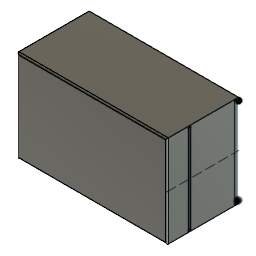
Control board - base v4 (Autodesk Fusion 360 design; units mm, degrees)
Autodesk Fusion 360 part; units mm, degrees
sketch "Esquisse1" plane through (0, 0, 0) normal (0, 1, 0) x (1, 0, 0)
  line L0 (-41.4317, -0.2961) -> (62.5683, -0.2961)
  line L1 (62.5683, -0.2961) -> (62.5683, -64.2961)
  line L2 (62.5683, -64.2961) -> (-41.4317, -64.2961)
  line L3 (-41.4317, -64.2961) -> (-41.4317, -0.2961)
  dimension "d1" = 104
  dimension "d2" = 64
  constraint horizontal L0
  constraint vertical L1
  constraint horizontal L2
  constraint vertical L3
  measures "d1" distance of L1 L3
  measures "d2" distance of L0 L2
extrude "Extrusion1" add sketch "Esquisse1" along normal blind 50
shell "Coque1" thickness 2 removed faces 1 at (-6.765, 50, 21.6294)
sketch "Sketch4" plane through (62.5683, 0, 0) normal (1, 0, 0) x (0, 1, 0)
  line L0 (0, 64.2961) -> (0, 0.2961)
  line L1 (0, 0.2961) -> (50, 0.2961)
  line L2 (50, 0.2961) -> (50, 64.2961)
  line L3 (50, 64.2961) -> (0, 64.2961)
  line L4 (0, 32.2961) -> (50, 32.2961) construction
  line L5 (15, 63.3961) -> (16.4, 63.3961)
  line L6 (16.4, 63.3961) -> (16.4, 1.1961)
  line L7 (16.4, 1.1961) -> (15, 1.1961)
  line L8 (15, 1.1961) -> (15, 63.3961)
  line L9 (48.8, 1.1961) -> (47.4, 1.1961)
  line L10 (47.4, 1.1961) -> (47.4, 63.3961)
  line L11 (47.4, 63.3961) -> (48.8, 63.3961)
  line L12 (48.8, 63.3961) -> (48.8, 1.1961)
  line L13 (48.8, 62.2961) -> (50, 62.2961)
  line L14 (48.8, 2.2961) -> (50, 2.2961)
  dimension "d19" = 1.4
  dimension "d20" = 1.4
  dimension "d55" = 31
  dimension "d66" = 0.9
  dimension "d67" = 2
  dimension "d79" = 15
  constraint midpoint L0 L4.start
  constraint midpoint L2 L4.end
  constraint horizontal L5
  constraint vertical L6
  constraint horizontal L7
  constraint vertical L8
  constraint symmetric L4 L5 L7
  constraint horizontal L9
  constraint vertical L10
  constraint horizontal L11
  constraint vertical L12
  constraint symmetric L4 L9 L11
  constraint collinear L5 L11
  constraint coincident L12 L13.start
  constraint coincident L2 L13.end
  constraint perpendicular L2 L13
  constraint symmetric L4 L13.start L14.start
  constraint symmetric L4 L13.end L14.end
  measures "d19" distance of L6.end L7.end
  measures "d20" distance of L9.start L9.end
  measures "d55" distance of L6 L10
  measures "d66" distance of L3 L5
  measures "d67" distance of L3 L13
  measures "d79" distance of L0 L8
extrude "Extrude4" cut sketch "Sketch4" against normal blind 103.1 contours L9 L10 L11 L12 | L5 L6 L7 L8
sketch "Sketch8" plane through (0, 50, 0) normal (0, 1, 0) x (-1, 0, 0)
  line L0 (39.4317, 2.2961) -> (-60.5683, 2.2961)
  line L1 (-60.5683, 62.2961) -> (39.4317, 62.2961)
  line L2 (41.4317, 64.2961) -> (-62.5683, 64.2961)
  line L3 (-62.5683, 64.2961) -> (-62.5683, 0.2961)
  line L4 (-62.5683, 0.2961) -> (41.4317, 0.2961)
  line L5 (41.4317, 0.2961) -> (41.4317, 64.2961)
  line L6 (-60.5683, 2.2961) -> (-62.5683, 2.2961)
  line L7 (-62.5683, 2.2961) -> (-62.5683, 42.2961)
  line L8 (-60.5683, 42.2961) -> (-60.5683, 2.2961)
  line L9 (39.4317, 62.2961) -> (39.4317, 2.2961)
  line L10 (-60.5683, 2.2961) -> (-60.5683, 62.2961)
  line L11 (-60.5683, 62.2961) -> (-62.5683, 62.2961)
  line L12 (-60.5683, 42.2961) -> (-60.5683, 62.2961)
  line L13 (-62.5683, 42.2961) -> (-62.5683, 2.2961)
  constraint horizontal L6
  constraint vertical L7
  constraint vertical L8
  constraint coincident L0.end L6.start
  constraint coincident L1.start L10.end
  constraint coincident L3 L11.end
  constraint perpendicular L3 L11
extrude "Extrude6" cut sketch "Sketch8" against normal blind 1.3 contours L3 L6 L7 L8 L10 L11 L12 L13
sketch "Sketch9" plane through (0, 0, 64.2961) normal (0, 0, 1) x (-1, 0, 0)
  line L0 (-62.5683, 0) -> (-62.5683, -50)
  line L1 (-62.5683, -50) -> (41.4317, -50)
  line L2 (41.4317, -50) -> (41.4317, 0)
  line L3 (-62.5683, -45.1) -> (41.4317, -45.1) construction
  line L4 (-18.0683, -43.6) -> (-3.0683, -43.6)
  line L5 (-3.0683, -43.6) -> (-3.0683, -46.6)
  line L6 (-3.0683, -46.6) -> (-18.0683, -46.6)
  line L7 (-18.0683, -46.6) -> (-18.0683, -43.6)
  line L8 (-10.5683, -50) -> (-10.5683, -31.2) construction
  line L9 (41.4317, 0) -> (-62.5683, 0)
  dimension "d61" = 4.9
  dimension "d62" = 15
  dimension "d63" = 3
  constraint coincident L0 L3.start
  constraint coincident L2 L3.end
  constraint perpendicular L2 L3
  constraint horizontal L4
  constraint vertical L5
  constraint horizontal L6
  constraint vertical L7
  constraint symmetric L3 L4 L6
  constraint midpoint L1 L8.start
  constraint symmetric L5 L7 L8
  measures "d61" distance of L1 L3
  measures "d62" distance of L4.start L4.end
  measures "d63" distance of L4.end L5.end
fillet "Fillet1" radius 1 4 edges at (10.5683, 0, 64.2961) (62.5683, 0, 32.2961) (10.5683, 0, 0.2961) (-41.4317, 0, 32.2961)
sketch "Sketch12" plane through (-41.4317, 0, 0) normal (-1, 0, 0) x (0, -1, 0)
  line L0 (-1, 0.2961) -> (-1, 64.2961)
  line L1 (-1, 64.2961) -> (-50, 64.2961)
  line L2 (-50, 64.2961) -> (-50, 0.2961)
  line L3 (-50, 0.2961) -> (-1, 0.2961)
  line L4 (-41.0361, 37.2961) -> (-36.0361, 37.2961)
  line L5 (-36.0361, 37.2961) -> (-36.0361, 27.2961)
  line L6 (-36.0361, 27.2961) -> (-41.0361, 27.2961)
  line L7 (-41.0361, 27.2961) -> (-41.0361, 37.2961)
  line L8 (-1, 32.2961) -> (-50, 32.2961) construction
  dimension "d80" = 5
  dimension "d81" = 10
  constraint horizontal L4
  constraint vertical L5
  constraint horizontal L6
  constraint vertical L7
  constraint midpoint L0 L8.start
  constraint midpoint L2 L8.end
  constraint symmetric L4 L6 L8
  measures "d80" distance of L4.start L4.end
  measures "d81" distance of L4.start L6.end
extrude "Extrude10" cut sketch "Sketch12" against normal blind 15 contours L4 L5 L6 L7
